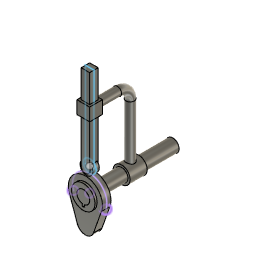
New_mech v1 (Autodesk Fusion 360 design; units mm, degrees)
Autodesk Fusion 360 part; units mm, degrees
note: some values were not read from the file. Set by a fixed rule: which sketch regions a step uses.
sketch "Sketch1" plane through (0, 0, 0) normal (0, 1, 0) x (1, 0, 0) in component "Cam"
  circle A0 centre (0, 0) radius 27.5
  circle A1 centre (0, 0) radius 40
  circle A2 centre (0, 60) radius 20
  line L0 (-37.7124, 13.3333) -> (-18.8562, 66.6667)
  line L1 (37.7124, 13.3333) -> (18.8562, 66.6667)
  line L2 (2.5, 20) -> (-2.5, 20)
  line L3 (-2.5, 20) -> (-2.5, 14.7902)
  line L4 (2.5, 14.7902) -> (2.5, 20)
  arc A3 (-2.5, -14.7902) -> (2.5, 14.7902) centre (0, 0) ccw
  arc A4 (-2.5, 14.7902) -> (-2.5, -14.7902) centre (0, 0) ccw
  dimension "d1" = 30
  dimension "d2" = 55
  dimension "d3" = 80
  dimension "d4" = 40
  dimension "d5" = 60
  constraint coincident A0.centre A1.centre
  constraint concentric A0 A3
  constraint coincident A1 L0.start
  constraint coincident A2 L0.end
  constraint tangent A2 L0
  constraint tangent A1 L0
  constraint horizontal L2
  constraint perpendicular L2 L3
  constraint coincident A3.start L3
  constraint coincident L3.end A3
  constraint concentric A3 A4
  measures "d1" diameter of A3
  measures "d2" diameter of A0
  measures "d3" diameter of A1
  measures "d4" diameter of A2
  measures "d5" distance of A0.centre A2.centre
extrude "Extrude1" add sketch "Sketch1" along normal mid plane 20 contours A1 | A1 A2 L1 | A1 A2 L0 | A2 makes body 1 in component "Cam"
extrude "Extrude2" add sketch "Sketch1" along normal mid plane 30 separate body contours A0 makes body 2 in component "Cam"
sketch "Sketch1 (2)" plane through (0, 0, 0) normal (0, 1, 0) x (1, 0, 0) in component "Follower"
  arc A0 (-37.7124, 13.3333) -> (37.7124, 13.3333) centre (0, 0) ccw
  circle A1 centre (0, -55) radius 15
  line L0 (10, -55) -> (10, -255)
  line L1 (10, -255) -> (-10, -255)
  line L2 (-10, -255) -> (-10, -55)
  arc A2 (10, -55) -> (-10, -55) centre (0, -55) ccw
  dimension "d14" = 30
  dimension "d15" = 20
  dimension "d16" = 20
  dimension "d17" = 200
  constraint concentric A1 A2
  constraint vertical L0
  constraint horizontal L1
  constraint vertical L2
  measures "d14" diameter of A1
  measures "d15" diameter of A2
  measures "d16" distance of L2.end L0.start
  measures "d17" distance of L2.end L1.end
extrude "Extrude6" add sketch "Sketch1 (2)" along normal mid plane 15 separate body contours A1 L0 L2 A2 | A1 L0 L2 A2 makes body 3 in component "Follower"
extrude "Extrude7" add sketch "Sketch1 (2)" along normal mid plane 20 separate body contours A1 L0 L1 L2 | A1 L0 L2 A2 picked at (0, -60) makes body 4 in component "Follower"
combine "Combine1" operation cut target body 4 tool bodies 3 keep tools in component "Follower"
sketch "Sketch1 (3)" plane through (0, -15, 0) normal (0, -1, 0) x (1, 0, 0) in component "Shaft"
  arc A0 (2.5, -14.7902) -> (-2.5, -14.7902) centre (0, 0) ccw
  line L0 (2.5, -14.7902) -> (2.5, -20)
  line L1 (2.5, -20) -> (-2.5, -20)
  line L2 (-2.5, -20) -> (-2.5, -14.7902)
  circle A1 centre (0, 0) radius 27.5
extrude "Extrude1'" add sketch "Sketch1 (3)" against normal blind 30 separate body contours A0 L0 L1 L2 makes body 5 in component "Shaft"
cylinder "CylinderPrimitive1" add diameter 30 height 180 placed x (1, 0, 0) y (0, 0, -1) z (0, 1, 0) at (0, 15, 0) bodies 5 in component "Shaft"
sketch "Sketch1 (4)" plane through (0, 0, 0) normal (1, 0, 0) x (0, 1, 0) in component "Base"
  line L0 (195, -15) -> (195, 15)
  line L1 (-15, -20) -> (-15, -14.7902)
  line L2 (15, -20) -> (15, -15)
  line L3 (-15, -20) -> (15, -20)
  line L4 (-15, 15) -> (-15, -14.7902)
  line L5 (15, -15) -> (195, -15)
  line L6 (-15, 15) -> (195, 15)
  line L7 (75, 15) -> (115, 15)
  line L8 (115, 15) -> (115, 20)
  line L9 (115, 20) -> (75, 20)
  line L10 (75, 20) -> (75, 15)
  line L11 (15, -27.5) -> (15, 27.5)
  line L12 (95, 15) -> (95, 145)
  line L13 (65, 175) -> (15, 175)
  arc A0 (95, 145) -> (65, 175) centre (65, 145) ccw
  point P0 (95, 175)
  dimension "d36" = 40
  dimension "d37" = 5
  dimension "d38" = 60
  dimension "d39" = 160
  dimension "d40" = 80
  dimension "d41" = 30
  constraint horizontal L7
  constraint vertical L8
  constraint horizontal L9
  constraint vertical L10
  constraint coincident L6 L7.start
  constraint midpoint L7 L12.start
  constraint perpendicular L7 L12
  constraint perpendicular L12 L13
  constraint coincident P0 L12
  constraint coincident P0 L13
  constraint tangent L12 A0
  constraint tangent L13 A0
  measures "d36" distance of L7.start L7.end
  measures "d37" distance of L7.start L9.end
  measures "d38" distance of L7.start L11
  measures "d39" distance of L12.start P0
  measures "d40" distance of P0 L13.end
  measures "d41" radius of A0
revolve "Revolve1" add sketch "Sketch1 (4)" angle 360 about axis through (0, -15, 0) along (0, -1, 0) separate body contours L6 L7 L8 L9 L12 | L6 L7 L9 L10 L12 makes body 6 in component "Base"
pipe "Pipe1" add diameter 20 path "Sketch1 (4)" along L12 A0 L13 separate body makes body 7 in component "Base"
ref_plane "WorkPlane1" through (0, 40, 175) normal (0, 0, 1) x (0, -1, 0) in component "Base"
sketch "Sketch2" plane through (0, 0, 175) normal (0, 0, 1) x (1, 0, 0) in component "Base"
  line L0 (10, -7.5) -> (10, 7.5)
  line L1 (-10, 7.5) -> (-10, -7.5)
  line L2 (-10, -10) -> (-10, -7.5)
  line L3 (-10, 7.5) -> (-10, 10)
  line L4 (10, -10) -> (10, -7.5)
  line L5 (-10, -10) -> (10, -10)
  line L6 (10, 10) -> (-10, 10)
  line L7 (10, 7.5) -> (10, 10)
  line L8 (-15, 7.5) -> (-15, 15)
  line L9 (15, 15) -> (-15, 15)
  line L10 (15, 7.5) -> (15, 15)
  line L11 (15, -7.5) -> (15, 7.5)
  line L12 (15, -15) -> (15, -7.5)
  line L13 (-15, -15) -> (15, -15)
  line L14 (-15, -15) -> (-15, -7.5)
  line L15 (-15, 7.5) -> (-15, -7.5)
  dimension "d48" = 5
extrude "Extrude1''" add sketch "Sketch2" along normal mid plane 30 bodies 7 in component "Base"
combine "Combine1'" operation add target body 7 tool bodies 6 in component "Base"
component "Cam" placed x (1, 0, 0) y (0, 1, 0) z (0, 0, 1) at (0, 0, 0)
component "Shaft" placed x (1, 0, 0) y (0, 1, 0) z (0, 0, 1) at (0, 0, 0)
component "Follower" placed x (1, 0, 0) y (0, 1, 0) z (0, 0, 1) at (0, 0, 0)
component "Base" placed x (1, 0, 0) y (0, 1, 0) z (0, 0, 1) at (0, 0, 0)
